Autodesk Fusion 360 part; units mm, degrees
(part 2 of 2)
sketch "Sketch15" plane through (190.1478, 0, 0) normal (-1, 0, 0) x (0, -1, 0)
  line L0 (175.5481, -2) -> (135.5481, -2)
  line L1 (135.5481, -2) -> (135.5481, -17)
  line L2 (135.5481, -17) -> (175.5481, -17)
  line L3 (175.5481, -17) -> (175.5481, -2)
  line L4 (155.5481, -17) -> (155.5481, -2) construction
  line L5 (135.5481, -2) -> (155.5481, -17) construction
  line L6 (155.5481, -17) -> (175.5481, -2) construction
  circle A0 centre (165.5481, -9.5) radius 2
  circle A1 centre (145.5481, -9.5) radius 2
  dimension "d205" = 4
  dimension "d206" = 4
  constraint midpoint L2 L4.start
  constraint midpoint L0 L4.end
  constraint coincident L0.end L1.start
  constraint coincident L0.start L3.end
  constraint midpoint L6 A0.centre
  constraint midpoint L5 A1.centre
  measures "d205" diameter of A0
  measures "d206" diameter of A1
extrude "Extrude20" cut sketch "Sketch15" against normal blind 4 contours A0 | A1 bodies 5
sketch "Sketch16" plane through (190.1478, 0, 0) normal (-1, 0, 0) x (0, -1, 0)
  line L0 (68.4519, -2) -> (28.4519, -2)
  line L1 (28.4519, -2) -> (28.4519, -17)
  line L2 (28.4519, -17) -> (68.4519, -17)
  line L3 (68.4519, -17) -> (68.4519, -2)
  line L4 (48.4519, -17) -> (48.4519, -2) construction
  line L5 (48.4519, -17) -> (28.4519, -2) construction
  arc A0 (48.4519, -17) -> (49.0226, -16.239) centre (48.7373, -16.6195) ccw construction
  line L6 (49.0226, -16.239) -> (68.4519, -2) construction
  circle A1 centre (38.4519, -9.5) radius 2
  circle A2 centre (58.7373, -9.1195) radius 2
  dimension "d209" = 4
  dimension "d210" = 4
  constraint midpoint L2 L4.start
  constraint midpoint L0 L4.end
  constraint coincident L0.end L1.start
  constraint tangent L5 A0
  constraint coincident L0.start L3.end
  constraint midpoint L5 A1.centre
  constraint midpoint L6 A2.centre
  measures "d209" diameter of A1
  measures "d210" diameter of A2
extrude "Extrude21" cut sketch "Sketch16" against normal blind 4 contours A1 | A2 bodies 5
sketch "Sketch17" plane through (0, 0, -2) normal (0, 0, -1) x (1, 0, 0)
  line L0 (194.1478, 28.4519) -> (190.1478, 28.4519)
  line L1 (190.1478, 28.4519) -> (190.1478, 68.4519)
  line L2 (190.1478, 68.4519) -> (194.1478, 68.4519)
  line L3 (194.1478, 68.4519) -> (194.1478, 28.4519)
  line L4 (190.1478, 135.5481) -> (190.1478, 175.5481)
  line L5 (190.1478, 175.5481) -> (194.1478, 175.5481)
  line L6 (194.1478, 175.5481) -> (194.1478, 135.5481)
  line L7 (194.1478, 135.5481) -> (190.1478, 135.5481)
  circle A0 centre (13.1491, 10.9445) radius 2.5
  arc A1 (71.1448, 62.4445) -> (73.6448, 59.9447) centre (71.1448, 59.9445) ccw
  line L8 (71.1448, 62.4445) -> (13.1478, 62.4445)
  circle A2 centre (13.1491, 59.9445) radius 2.5
  line L9 (13.1478, 62.4445) -> (13.1478, 178)
  line L10 (13.1478, 178) -> (179.1478, 178)
  line L11 (179.1478, 178) -> (179.1478, 26)
  line L12 (179.1478, 26) -> (73.6478, 26)
  line L13 (73.6478, 26) -> (73.6448, 59.9447)
  line L14 (205.1478, 26.0329) -> (205.1478, 177.9671)
  line L15 (205.1478, 177.9671) -> (371.1478, 177.9671)
  line L16 (371.1478, 177.9671) -> (371.1478, 26.0329)
  line L17 (371.1478, 26.0329) -> (205.1478, 26.0329)
  arc A3 (380.935, 102.943) -> (384.4722, 101.0754) centre (382.7081, 102.0177) ccw
  arc A4 (384.4722, 101.0754) -> (380.935, 102.943) centre (382.6992, 102.0007) ccw
  arc A5 (198.1079, 103.9615) -> (198.3492, 99.9688) centre (198.233, 101.9654) ccw
  arc A6 (198.3492, 99.9688) -> (198.1079, 103.9615) centre (198.2241, 101.9648) ccw
  circle A7 centre (186.0715, 101.9648) radius 2
  circle A8 centre (1.5965, 102.0007) radius 2
  circle A9 centre (96.15, 193) radius 2
  circle A10 centre (96.1478, 10.9519) radius 2
  line L18 (388.744, 209.0962) -> (-4.4484, 209.0962)
  arc A11 (-4.4484, 209.0962) -> (-10.9305, 202.1145) centre (-4.4484, 202.5962) ccw
  line L19 (-10.9305, 202.1145) -> (-10.9394, 102)
  line L20 (-10.9394, 102) -> (-10.9305, 1.8855)
  arc A12 (-10.9305, 1.8855) -> (-4.4484, -5.0962) centre (-4.4484, 1.4038) ccw
  line L21 (-4.4484, -5.0962) -> (388.744, -5.0962)
  arc A13 (388.744, -5.0962) -> (395.244, 1.4038) centre (388.744, 1.4038) ccw
  line L22 (395.244, 1.4038) -> (395.244, 202.5962)
  arc A14 (395.244, 202.5962) -> (388.744, 209.0962) centre (388.744, 202.5962) ccw
  arc A15 (286.156, 193.2036) -> (290.1361, 192.8049) centre (288.1465, 193.0085) ccw
  arc A16 (290.1361, 192.8049) -> (286.156, 193.2036) centre (288.1456, 193) ccw
  arc A17 (287.2606, 12.7444) -> (289.0521, 9.168) centre (288.1649, 10.9605) ccw
  arc A18 (289.0521, 9.168) -> (287.2606, 12.7444) centre (288.1478, 10.9519) ccw
  circle A19 centre (71.1491, 10.9445) radius 2.5
  circle A20 centre (-4.4484, 202.5962) radius 5.5
  circle A21 centre (388.744, 202.5962) radius 5.5
  circle A22 centre (388.744, 1.4038) radius 5.5
  circle A23 centre (-4.4484, 1.4038) radius 5.5
  line L23 (-9.9484, 1.4038) -> (-9.9484, 202.5962)
  line L24 (-4.4484, 208.0962) -> (388.744, 208.0962)
  line L25 (394.244, 202.5962) -> (394.244, 1.4038)
  line L26 (388.744, -4.0962) -> (-4.4484, -4.0962)
  dimension "d213" = 11
  dimension "d214" = 11
  dimension "d215" = 11
  dimension "d216" = 11
  constraint concentric A11 A20
  constraint concentric A14 A21
  constraint concentric A13 A22
  constraint concentric A12 A23
  constraint coincident A23 L23.start
  constraint coincident A20 L23.end
  constraint tangent A20 L23
  constraint vertical L23
  constraint coincident A20 L24.start
  constraint coincident A21 L24.end
  constraint tangent A21 L24
  constraint perpendicular L23 L24
  constraint coincident A21 L25.start
  constraint coincident A22 L25.end
  constraint tangent A22 L25
  constraint perpendicular L24 L25
  constraint coincident A22 L26.start
  constraint coincident A23 L26.end
  constraint tangent A23 L26
  constraint perpendicular L25 L26
  measures "d213" diameter of A20
  measures "d214" diameter of A21
  measures "d215" diameter of A22
  measures "d216" diameter of A23
extrude "Extrude22" add sketch "Sketch17" along normal blind 25 contours L18 A11 L19 L20 A12 L21 A13 L22 A14 bodies 5
sketch "Sketch18" plane through (-10.9304, 0.001, 0) normal (-1, 0.000089, 0) x (-0.000089, -1, 0)
  line L0 (102.001, 0) -> (1.8864, 0)
  line L1 (1.8864, 0) -> (1.8864, -27)
  line L2 (1.8864, -27) -> (102.001, -27)
  line L3 (102.001, -27) -> (102.001, 0)
  circle A0 centre (4.6364, -27) radius 2.75
  dimension "d219" = 5.5
  constraint coincident L1.end A0
  measures "d219" diameter of A0
extrude "Extrude23" cut sketch "Sketch18" against normal blind 2 contours L2 A0 picked at (5.5124, -26.7298) bodies 5
equation "d16 = ( 192 * 2 ) * 1 mm"
equation "d87 = ( 192 * 2 ) * 1 mm"
equation "d139 = ( 192 * 2 ) * 1 mm"
